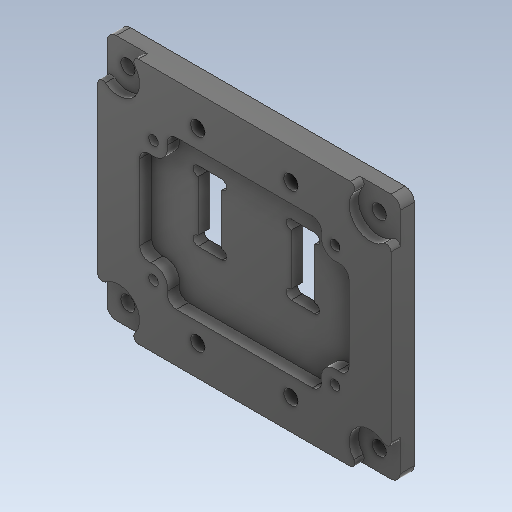
# Autodesk Inventor part: Camera_horizontal_frame_01
Saved by Autodesk Inventor 2020.4 (Build 244396000, 396)
## iProperties
Created: 2021-08-26
Part Number: Camera_horizontal_frame_01
Material: アセタール樹脂、黒
Document SubType Name: Modeling
Designer: t-nagamine
Density: 1.425 g/cm^3
Appearance: 滑らか - 黒
Description: POM T5
Author: t-nagamine
Autodesk Inventor part; units mm, degrees
ref_plane "YZ Plane" through (0, 0, 0) normal (1, 0, 0) x (0, 1, 0)
ref_plane "XZ Plane" through (0, 0, 0) normal (0, 1, 0) x (-1, 0, 0)
ref_plane "XY Plane" through (0, 0, 0) normal (0, 0, 1) x (1, 0, 0)
derived "Camera_cover_01.ipt"
sketch "スケッチ1" plane through (0, 0, 0) normal (0, 0, 1) x (1, 0, 0)
  line L0 (-37, 32) -> (37, 32)
  line L1 (37, 32) -> (37, -32)
  line L2 (37, -32) -> (-37, -32)
  line L3 (-37, -32) -> (-37, 32)
  line L4 (-37, 32) -> (37, -32) construction
  line L5 (37, 32) -> (-37, -32) construction
  line L6 (-32, 27) -> (32, 27)
  line L7 (32, 27) -> (32, -27)
  line L8 (32, -27) -> (-32, -27)
  line L9 (-32, -27) -> (-32, 27)
  line L10 (-32, 27) -> (32, -27) construction
  line L11 (32, 27) -> (-32, -27) construction
  arc A0 (-30, 27) -> (-32, 25) centre (-30, 25) ccw
  line L12 (0, 32) -> (0, -32) construction
  line L13 (37, 0) -> (-37, 0) construction
  arc A1 (-32, -25) -> (-30, -27) centre (-30, -25) ccw
  arc A2 (32, 25) -> (30, 27) centre (30, 25) ccw
  arc A3 (30, -27) -> (32, -25) centre (30, -25) ccw
  circle A4 centre (-27, 22) radius 2
  circle A5 centre (-27, 22) radius 4
  line L14 (-32, 21.3431) -> (-29.8284, 19.1716)
  line L15 (-26.3431, 27) -> (-24.1716, 24.8284)
  circle A6 centre (-27, -22) radius 4
  circle A7 centre (-27, -22) radius 2
  line L16 (-26.3431, -27) -> (-24.1716, -24.8284)
  line L17 (-32, -21.3431) -> (-29.8284, -19.1716)
  line L18 (32, 27) -> (-32, -27) construction
  circle A8 centre (27, 22) radius 4
  circle A9 centre (27, 22) radius 2
  line L19 (26.3431, 27) -> (24.1716, 24.8284)
  line L20 (32, 21.3431) -> (29.8284, 19.1716)
  circle A10 centre (27, -22) radius 4
  circle A11 centre (27, -22) radius 2
  line L21 (32, -21.3431) -> (29.8284, -19.1716)
  line L22 (26.3431, -27) -> (24.1716, -24.8284)
  circle A12 centre (0, 0) radius 8
  line L23 (-32, 10) -> (-37, 10)
  line L24 (-32, -10) -> (-37, -10)
  line L25 (24, 15) -> (-24, 15)
  line L26 (-24, 15) -> (-24, -15)
  line L27 (-24, -15) -> (24, -15)
  line L28 (24, -15) -> (24, 15)
  line L29 (24, 15) -> (-24, -15) construction
  line L30 (-24, 15) -> (24, -15) construction
  line L31 (24, 10) -> (19, 15)
  line L32 (24, -10) -> (19, -15)
  line L33 (-24, 10) -> (-19, 15)
  line L34 (-24, -10) -> (-19, -15)
  line L35 (-31.5, 26.5) -> (31.5, 26.5)
  line L36 (31.5, 26.5) -> (31.5, -26.5)
  line L37 (31.5, -26.5) -> (-31.5, -26.5)
  line L38 (-31.5, -26.5) -> (-31.5, 26.5)
  line L39 (-31.5, 26.5) -> (31.5, -26.5) construction
  line L40 (31.5, 26.5) -> (-31.5, -26.5) construction
  arc A13 (-29.5, 26.5) -> (-31.5, 24.5) centre (-29.5, 24.5) ccw
  arc A14 (31.5, 24.5) -> (29.5, 26.5) centre (29.5, 24.5) ccw
  arc A15 (-31.5, -24.5) -> (-29.5, -26.5) centre (-29.5, -24.5) ccw
  arc A16 (29.5, -26.5) -> (31.5, -24.5) centre (29.5, -24.5) ccw
  circle A17 centre (-27, 22) radius 1.55
  circle A18 centre (27, 22) radius 1.55
  circle A19 centre (-27, -22) radius 1.55
  circle A20 centre (27, -22) radius 1.55
  line L41 (-22.5, 16) -> (22.5, 16)
  line L42 (22.5, 16) -> (22.5, -16)
  line L43 (22.5, -16) -> (-22.5, -16)
  line L44 (-22.5, -16) -> (-22.5, 16)
  line L45 (-22.5, 16) -> (22.5, -16) construction
  line L46 (22.5, 16) -> (-22.5, -16) construction
  circle A21 centre (-19.5, 13) radius 3
  circle A22 centre (-19.5, 13) radius 1.05
  circle A23 centre (19.5, 13) radius 3
  circle A24 centre (19.5, 13) radius 1.05
  circle A25 centre (-19.5, -13) radius 3
  circle A26 centre (-19.5, -13) radius 1.05
  circle A27 centre (19.5, -13) radius 3
  circle A28 centre (19.5, -13) radius 1.05
  line L47 (-12.55, 10.55) -> (-7.45, 10.55)
  line L48 (-12.55, 8.45) -> (-12.55, -2.45)
  arc A29 (-12.55, 10.55) -> (-12.55, 8.45) centre (-12.55, 9.5) ccw
  line L49 (-7.45, 8.45) -> (-7.45, -2.45)
  arc A30 (-7.45, 8.45) -> (-7.45, 10.55) centre (-7.45, 9.5) ccw
  line L50 (-12.55, -4.55) -> (-7.45, -4.55)
  arc A31 (-12.55, -2.45) -> (-12.55, -4.55) centre (-12.55, -3.5) ccw
  arc A32 (-7.45, -4.55) -> (-7.45, -2.45) centre (-7.45, -3.5) ccw
  line L51 (12.55, 10.55) -> (7.45, 10.55)
  line L52 (12.55, 8.45) -> (12.55, -2.45)
  arc A33 (12.55, 8.45) -> (12.55, 10.55) centre (12.55, 9.5) ccw
  line L53 (7.45, 8.45) -> (7.45, -2.45)
  arc A34 (7.45, 10.55) -> (7.45, 8.45) centre (7.45, 9.5) ccw
  line L54 (12.55, -4.55) -> (7.45, -4.55)
  arc A35 (12.55, -4.55) -> (12.55, -2.45) centre (12.55, -3.5) ccw
  arc A36 (7.45, -2.45) -> (7.45, -4.55) centre (7.45, -3.5) ccw
  circle A37 centre (-27, 22) radius 4.5
  line L55 (-31.5, 20.136) -> (-30.182, 18.818)
  line L56 (-25.136, 26.5) -> (-23.818, 25.182)
  circle A38 centre (27, 22) radius 4.5
  line L57 (31.5, 20.136) -> (30.182, 18.818)
  line L58 (25.136, 26.5) -> (23.818, 25.182)
  circle A39 centre (-27, -22) radius 4.5
  line L59 (-31.5, -20.136) -> (-30.182, -18.818)
  line L60 (-25.136, -26.5) -> (-23.818, -25.182)
  line L61 (25.136, -26.5) -> (23.818, -25.182)
  circle A40 centre (27, -22) radius 4.5
  line L62 (31.5, -20.136) -> (30.182, -18.818)
  circle A41 centre (-10, 20) radius 1.55
  circle A42 centre (10, 20) radius 1.55
  circle A43 centre (-10, -20) radius 1.55
  circle A44 centre (10, -20) radius 1.55
  line L63 (32, -10) -> (37, -10)
  line L64 (32, 27) -> (32, 32)
  point P0 (-31.5, -24.5)
  point P1 (31.5, -24.5)
  point P2 (31.5, 24.5)
  point P3 (22.5, -13)
  point P4 (22.5, 13)
  point P5 (19.5, 16)
  point P6 (-19.5, 16)
  point P7 (-22.5, 13)
  point P8 (-22.5, -13)
  point P9 (-19.5, -16)
  point P10 (19.5, -16)
  point P11 (25.8431, -26.5)
  point P12 (31.5, -20.8431)
  point P13 (31.5, 20.8431)
  point P14 (25.8431, 26.5)
  point P15 (-25.8431, 26.5)
  point P16 (-31.5, 20.8431)
  point P17 (-31.5, -20.8431)
  point P18 (-25.8431, -26.5)
  point P19 (10.0149, -4.55)
  point P20 (-10.0149, -4.55)
  point P21 (-7.45, 2.915)
  point P22 (7.45, 2.915)
  point P23 (17.2639, -15)
  point P24 (22.2343, -11.7657)
  point P25 (22.5, -11.5)
  point P26 (22.5, 11.5)
  point P27 (22.2343, 11.7657)
  point P28 (17.2639, 15)
  point P29 (-17.2639, 15)
  point P30 (-22.2343, 11.7657)
  point P31 (-22.5, 11.5)
  point P32 (-22.5, -11.5)
  point P33 (-22.2343, -11.7657)
  point P34 (-17.2639, -15)
  point P35 (-6.7546, -4.2867)
  point P36 (6.7546, -4.2867)
  dimension "d1" = 63
  dimension "d2" = 53
  dimension "d3" = 2
  dimension "d4" = 2
  dimension "d5" = 2
  dimension "d11" = 3.1
  dimension "d12" = 45
  dimension "d13" = 32
  dimension "d14" = 6
  dimension "d15" = 2.1
  dimension "d19" = 5.1
  dimension "d20" = 10.55
  dimension "d21" = 12.55
  dimension "d26" = 10.9
  dimension "d27" = 12.55
  dimension "d28" = 2.1
  dimension "d29" = 10.9
  dimension "d30" = 5.1
  dimension "d31" = 2.1
  dimension "d35" = 5.1
  dimension "d36" = 4.55
  dimension "d37" = 12.55
  dimension "d56" = 9
  dimension "d58" = 45
  dimension "d59" = 45
  dimension "d64" = 3.1
  dimension "d65" = 6.5
  dimension "d66" = 21.5
  measures "d1" distance of L36.end L37.end
  measures "d2" distance of L35.end L36.end
  measures "d3" radius of A13
  measures "d4" distance of L35.start A13.start
  measures "d5" distance of L35.start A13.end
  measures "d11" diameter of A17
  measures "d12" distance of L42.end L43.end
  measures "d13" distance between parallel lines of L43 L41
  measures "d14" diameter of A21
  measures "d15" diameter of A22
  measures "d19" distance of L47.start L47.end
  measures "d20" distance between parallel lines of L13 L47
  measures "d21" distance from line of L12 L47.start
  measures "d26" distance of L48.start L48.end
  measures "d27" distance between parallel lines of L12 L48
  measures "d28" distance of L47.start L48.start
  measures "d29" distance of L49.start L49.end
  measures "d30" distance between parallel lines of L48 L49
  measures "d31" distance of L47.end L49.start
  measures "d35" distance of L50.start L50.end
  measures "d36" distance from line of L13 L50.start
  measures "d37" distance from line of L12 L50.start
  measures "d56" diameter of A37
  measures "d58" angle of L38 L55
  measures "d59" angle of L35 L56
  measures "d64" diameter of A41
  measures "d65" distance from line of L35 A41.centre
  measures "d66" distance from line of L38 A41.centre
extrude "押し出し1" add sketch "スケッチ1" against normal blind 5 contours L38 A37 L14 | L14 A37 L55 L38 | L35 A38 L19 | L19 A38 L58 L35 | A14 L36 A38 L35 | L36 L57 A38 L20 | L20 A38 L36 | L38 L59 A39 L17 | L17 A39 L38 | A37 L15 A5 L14 | L14 A5 L15 A37 | L55 A37 L56 L35 L58 A38 L57 L36 L62 A40 L61 L37 L60 A39 L59 L38 | L38 A13 L35 A37 | L36 A40 L21 | L21 A40 L62 L36 | L35 L56 A37 L15 | L15 A37 L35 | A38 L20 A8 L19 | L19 A8 L20 A38 | A39 L16 A6 L17 | L17 A6 L16 A39 | A39 L37 A15 L38 | A5 | A40 L22 A10 L21 | L21 A10 L22 A40 | L36 A16 L37 A40 | A8 | A6 | A39 L16 L37 | A10 | L37 L22 A40 | L16 A39 L60 L37 | A40 L22 L37 L61 | A4 | A7 | A9 | A11 | A12 A36 L53 | A12 L53 A34 L51 A33 L52 A35 L54 A36 | L53 A36 A12 A32 L49 | L49 A32 A12 | A12 A32 L50 A31 L48 A29 L47 A30 L49 | L28 L31 L42 L25 | L42 A23 L25 | L25 A23 L41 L42 | L28 L32 L42 L31 | A23 L31 L25 | L25 A23 | L42 L31 A23 | L28 L27 L42 L32 | L42 L32 A27 L27 A25 L34 L44 L33 A21 L25 A23 L31 | L31 A23 L25 | A23 L25 A21 L41 | L42 A27 L32 | A21 L25 L44 L41 | A21 L25 | L42 L43 A27 L27 | L27 A27 L42 | A27 L27 L32 | L32 L27 A27 | A21 L33 L25 | A21 L44 L25 | L25 L33 A21 | A27 L27 | A27 L43 A25 L27 | L44 L33 L26 L25 | A21 L33 L44 | A25 L27 | L27 L34 A25 | L44 L34 L26 L33 | L43 L44 L27 A25 | L27 A25 L34 | L44 L27 L26 L34 | L34 A25 L44 | L27 L44 A25 | A17 | A18 | A19 | A20 | A22 | A24 | A26 | A28 | A41 | A42 | A43 | A44
extrude "押し出し6" cut sketch "スケッチ1" against normal through all contours A17 | A18 | A19 | A20 | A22 | A24 | A26 | A28 | A41 | A42 | A43 | A44
extrude "押し出し7" cut sketch "スケッチ1" against normal blind 2.6 contours A12 A36 L53 | A12 L53 A34 L51 A33 L52 A35 L54 A36 | L53 A36 A12 A32 L49 | L49 A32 A12 | A12 A32 L50 A31 L48 A29 L47 A30 L49 | L42 L31 A23 | L42 L32 A27 L27 A25 L34 L44 L33 A21 L25 A23 L31 | A23 L25 A21 L41 | L42 A27 L32 | A27 L43 A25 L27 | A21 L33 L44 | L34 A25 L44
fillet "フィレット2" radius 2 8 edges at (-22.5, 13, -1.3) (-19.5, 16, -1.3) (22.5, 13, -1.3) (19.5, 16, -1.3) (19.5, -16, -1.3) (22.5, -13, -1.3) (-22.5, -13, -1.3) (-19.5, -16, -1.3)
extrude "押し出し8" cut sketch "スケッチ1" against normal through all contours A12 A36 L53 | A12 L53 A34 L51 A33 L52 A35 L54 A36 | L49 A32 A12 | A12 A32 L50 A31 L48 A29 L47 A30 L49
extrude "押し出し9" cut sketch "スケッチ1" against normal blind 2 contours L38 A37 L14 | L14 A37 L55 L38 | L35 A38 L19 | L19 A38 L58 L35 | A14 L36 A38 L35 | L36 L57 A38 L20 | L20 A38 L36 | L38 L59 A39 L17 | L17 A39 L38 | A37 L15 A5 L14 | L14 A5 L15 A37 | L38 A13 L35 A37 | L36 A40 L21 | L21 A40 L62 L36 | L35 L56 A37 L15 | L15 A37 L35 | A38 L20 A8 L19 | L19 A8 L20 A38 | A39 L16 A6 L17 | L17 A6 L16 A39 | A39 L37 A15 L38 | A5 | A40 L22 A10 L21 | L21 A10 L22 A40 | L36 A16 L37 A40 | A8 | A6 | A39 L16 L37 | A10 | L37 L22 A40 | L16 A39 L60 L37 | A40 L22 L37 L61 | A4 | A7 | A9 | A11 | A17 | A18 | A19 | A20
fillet "フィレット3" radius 1 8 edges at (25.136, 26.5, -1) (31.5, 20.136, -1) (31.5, -20.136, -1) (25.136, -26.5, -1) (-31.5, 20.136, -1) (-25.136, 26.5, -1) (-31.5, -20.136, -1) (-25.136, -26.5, -1)
